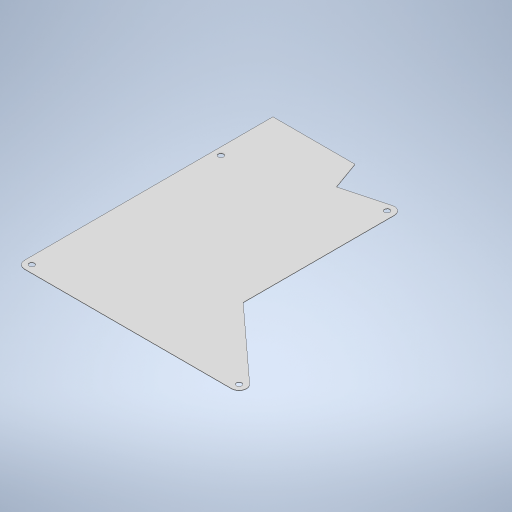
# Autodesk Inventor part: base_main_pcb_p2
Saved by Autodesk Inventor 2024 (Build 280153000, 153)
## iProperties
Created: 2026-03-21
Part Number: base_main_pcb_p2
Material: Generic
Document SubType Name: Modeling
Designer: schar
Density: 1 g/cm^3
Appearance: Default
Author: schar
Autodesk Inventor part; units mm, degrees
ref_plane "YZ Plane" through (0, 0, 0) normal (1, 0, 0) x (0, 1, 0)
ref_plane "XZ Plane" through (0, 0, 0) normal (0, 1, 0) x (-1, 0, 0)
ref_plane "Work Plane1" through (-197.5, 0.2, 285.96) normal (0, -1, 0) x (1, 0, 0)
sketch "Sketch1" plane through (-197.5, 0.2, 285.96) normal (0, -1, 0) x (1, 0, 0)
  line L0 (-4.5, -266.96) -> (-4.5, -4.5) projected
  line L1 (-4.5, -154.3852) -> (45.0203, -154.3852)
  line L2 (51.2973, -136.9464) -> (22.584, -216.7184) projected
  line L3 (45.0203, -154.3852) -> (51.2973, -136.9464)
  arc A0 (77.325, -143.9366) -> (83.5, -139.76) centre (79, -139.76) ccw projected
  line L4 (51.2973, -136.9464) -> (77.325, -143.9366)
  line L5 (83.5, -139.76) -> (83.5, -48.4312)
  arc A1 (128.2704, -7.591) -> (125, 0) centre (125, -4.5) ccw projected
  arc A2 (0, 0) -> (-4.5, -4.5) centre (0, -4.5) ccw projected
  line L6 (125, 0) -> (0, 0)
  line L7 (-4.5, -4.5) -> (-4.5, -154.3852)
  circle A3 centre (0, -4.5) radius 1.675 projected
  circle A4 centre (0, -4.5) radius 4.5
  circle A5 centre (79, -139.76) radius 1.675 projected
  circle A6 centre (79, -139.76) radius 4.5
  circle A7 centre (125, -4.5) radius 1.675 projected
  line L8 (128.2704, -7.591) -> (83.5, -48.4312) projected
  circle A8 centre (125, -4.5) radius 4.5
  line L9 (127.7784, -8.0399) -> (83.5, -48.4312)
  circle A9 centre (0, -118.51) radius 1.675 projected
  circle A10 centre (0, -118.51) radius 1.675
  circle A11 centre (5.9848, -142.4458) radius 2.5 projected
  circle A12 centre (5.9848, -142.4458) radius 2.5
  circle A13 centre (36.9406, -142.4458) radius 2.5 projected
  circle A14 centre (36.9406, -142.4458) radius 2.5
  point P0 (197.5, -285.96)
  constraints: 14 end point, 6 coincident, 4 centre point, 3 collinear, 2 horizontal, 2 horizontal alignment, 2 point on circle, 2 point on line, 1 tangent, 4 other
extrude "Extrusion1" add sketch "Sketch1" along normal blind 0.2 contours L0 A4 L6 A8 L8 L5 A6 L4 L2 L1 | A2 A4 | A1 L8 A8 | A6 A0 | A11 | A13
sketch "Sketch2" plane through (-197.5, 0, 285.96) normal (0, -1, 0) x (1, 0, 0)
  circle A0 centre (5.9848, -142.4458) radius 2.5 projected
  circle A1 centre (5.9848, -142.4458) radius 2.5
  circle A2 centre (36.9406, -142.4458) radius 2.5 projected
  circle A3 centre (36.9406, -142.4458) radius 2.5
  point P0 (197.5, -285.96)
  constraints: 2 centre point, 2 coincident
extrude "Extrusion2" add sketch "Sketch2" along normal blind 1
body "Solid2"
